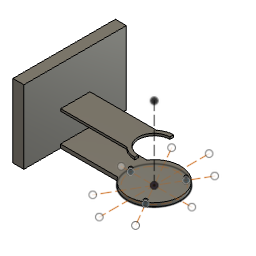
motor_support v1 (Autodesk Fusion 360 design; units mm, degrees)
Autodesk Fusion 360 part; units mm, degrees
sketch "스케치1" plane through (0, 0, 0) normal (0, 1, 0) x (1, 0, 0)
  circle A0 centre (0, 0) radius 36
  line L0 (-32.5898, 56.4472) -> (34.7247, -60.145) construction
  line L1 (0, 75) -> (0, -75) construction
  line L2 (51.4685, 0) -> (-45, 0) construction
  line L3 (30.2625, 52.4162) -> (-30.7015, -53.1766) construction
  circle A1 centre (0, 0) radius 32 construction
  circle A2 centre (16, -27.7128) radius 2.25
  circle A3 centre (16, 27.7128) radius 2.25
  circle A4 centre (-32, 0) radius 2.25
  line L4 (0, 0, 0) -> (0, 0, 100) construction
  point P0 (16, -27.7128)
  point P1 (16, 27.7128)
  point P2 (-32, 0)
  dimension "d2" = 72
  dimension "d3" = 30
  dimension "d4" = 30
  dimension "d5" = 64
  dimension "d6" = 4.5
  dimension "d29" = 100
  constraint coincident A0.centre A1.centre
  constraint coincident A0.centre L0
  constraint vertical L1
  constraint horizontal L2
  constraint coincident A0.centre L3
  constraint coincident A1 P0
  constraint coincident L0 P0
  constraint coincident L3 P1
  constraint coincident A1 P1
  constraint coincident A1 P2
  constraint coincident L2 P2
  constraint coincident P0 A2.centre
  constraint coincident P1 A3.centre
  constraint coincident P2 A4.centre
  constraint equal A2 A4
  constraint equal A2 A3
  measures "d2" diameter of A0
  measures "d3" angle of L0 L1
  measures "d4" angle of L1 L3
  measures "d5" diameter of A1
  measures "d6" diameter of A2
  measures "d29" distance of A0.centre A1.centre
extrude "돌출1" add sketch "스케치1" along normal blind 2
extrude "돌출2" add 1 faces at (0, 2, 0) along direction (0, 1, 0) blind 3
sketch "스케치2" plane through (0, 0, 0) normal (0, 1, 0) x (1, 0, 0)
  line L0 (20, -20) -> (-108, -20)
  line L1 (-108, -20) -> (-108, 20)
  line L2 (-108, 20) -> (20, 20)
  line L3 (20, 20) -> (20, -20)
  line L4 (0, 75) -> (0, -75)
  circle A0 centre (0, 0) radius 36
  line L5 (-108, -70) -> (-123, -70)
  line L6 (-123, -70) -> (-123, 70)
  line L7 (-123, 70) -> (-108, 70)
  line L8 (-108, 70) -> (-108, -70)
  dimension "d13" = 40
  dimension "d15" = 20
  dimension "d16" = 108
  dimension "d17" = 50
  dimension "d18" = 50
  dimension "d19" = 15
  constraint horizontal L0
  constraint vertical L1
  constraint horizontal L2
  constraint vertical L3
  constraint horizontal L5
  constraint vertical L6
  constraint horizontal L7
  constraint vertical L8
  constraint collinear L1 L8
  measures "d13" distance of L0.start L2.end
  measures "d15" distance of L3 L4
  measures "d16" distance of L1 A0.centre
  measures "d17" distance of L0 L5
  measures "d18" distance of L2 L7
  measures "d19" distance of L6 L8
extrude "돌출3" add sketch "스케치2" along normal blind 5 contours L0 L1 L2 A0 L8 | L1 L5 L6 L7 L8
extrude "돌출4" add sketch "스케치2" along normal blind 10 contours L1 L5 L6 L7 L8
extrude "돌출5" add 1 faces at (-113, 10, 23.3333) along direction (0, 1, 0) blind 15
extrude "돌출6" add 1 faces at (-113, 25, 23.3333) along direction (0, 1, 0) blind 75
ref_plane "작업 평면1" through (-43.5, 45, 0) normal (0, 1, 0) x (1, 0, 0)
sketch "스케치3" plane through (-36, 45, 0) normal (0, 1, 0) x (1, 0, 0)
  arc A0 (36, 21.5) -> (36, -21.5) centre (36, 0) ccw
  line L0 (36, 0, -45) -> (36, 0, 55)
  arc A1 (36, 26.5) -> (36, -26.5) centre (36, 0) ccw
  line L1 (36, 21.5) -> (36, 26.5)
  line L2 (36, -26.5) -> (36, -21.5)
  dimension "d30" = 21.5
  dimension "d31" = 5
  constraint coincident A0.centre A1.centre
  measures "d30" radius of A0
  measures "d31" distance of A0 A1
sketch "스케치5" plane through (-36, 45, 0) normal (0, 1, 0) x (1, 0, 0)
  line L0 (19.0243, 20.3488) -> (-72.2102, 20.3488)
  line L1 (-72.2102, 20.3488) -> (-72.2102, -19.6512)
  line L2 (-72.2102, -19.6512) -> (19.0243, -19.6512)
  arc A0 (36, 26.5) -> (36, -26.5) centre (36, 0) ccw
  line L3 (56, 20, -45) -> (56, -20, -45)
  constraint horizontal L0
  constraint vertical L1
  constraint horizontal L2
  constraint coincident L0.start A0
extrude "돌출7" add sketch "스케치3" sketch "스케치5" along normal blind 1.5 of sketch 2
extrude "돌출8" add 1 faces at (-79.1466, 45, -0.7681) along direction (0, -1, 0) blind 1.5
equation "d16 = 72 mm + 36 mm"
equation "d30 = ( 43 / 2 ) * 1 mm"
